Autodesk Inventor part; units mm, degrees
(part 2 of 2)
sketch "草圖23" plane through (-20, 166, 12) normal (0, 0, -1) x (-1, 0, 0)
  line L0 (0, 0) -> (1.75, 0)
  line L1 (9, 0) -> (0, 0) projected
  line L2 (1.75, 0) -> (7.25, 0)
  line L3 (7.25, 0) -> (9, 0)
  line L4 (1.75, 0) -> (7.25, 0)
  line L5 (7.25, 0) -> (7.25, 1)
  line L6 (7.25, 1) -> (1.75, 1)
  line L7 (1.75, 1) -> (1.75, 0)
  line L8 (1.75, 1) -> (7.25, 1)
  line L9 (7.25, 1) -> (7.25, 230)
  line L10 (1.75, 230) -> (1.75, 1)
  line L11 (7.25, 230) -> (7.25, 230.25)
  line L12 (7.25, 230.25) -> (1.75, 230.25)
  line L13 (1.75, 230.25) -> (1.75, 230)
  line L14 (1.75, 230) -> (2, 230)
  line L15 (7.25, 230) -> (7, 230)
  arc A0 (2, 230.25) -> (1.75, 230) centre (2, 230) ccw
  arc A1 (7.25, 230) -> (7, 230.25) centre (7, 230) ccw
  arc A2 (5.2071, 230.25) -> (3.7929, 230.25) centre (4.5, 230) ccw
  line L16 (7.25, 230) -> (5.25, 230)
  line L17 (2.25, 230) -> (1.75, 230)
  line L18 (1.75, 230) -> (3.75, 230)
  line L19 (6.75, 230) -> (7.25, 230)
  point P0 (-20, -166)
  dimension "d366" = 1.75
  dimension "d367" = 5.5
  dimension "d368" = 1
  dimension "d369" = 229
  dimension "d370" = 0.25
  dimension "d371" = 0.25
  dimension "d372" = 0.25
  dimension "d373" = 1.5
  constraints: 38 end point, 10 point on circle, 8 parallel, 8 point on line, 6 collinear, 4 perpendicular, 3 centre point, 2 coincident, 1 horizontal, 1 midpoint, 1 tangent
  measures "d366" distance of L0.start L0.end
  measures "d367" distance of L0.end L2.end
  measures "d368" distance of L5.end L2.end
  measures "d369" distance of L9.end L5.end
  measures "d370" distance of L11.end L9.end
  measures "d371" distance of L10.start L14.end
  measures "d372" distance of L9.end L15.end
  measures "d373" diameter of A2
extrude "擠出20" cut sketch "草圖23" against normal blind 0.6 contours L6 L10 A0 L12 A1 L9 | L12 A2
chamfer "倒角1" distance 3.2 angle 45 8 edges at (-20, 467.5, 28.5) (-20, 484.5, 24.5) (20, 484.5, 24.5) (20, 467.5, 28.5) (-20, 467.5, -28.5) (-20, 484.5, -24.5) (20, 484.5, -24.5) (20, 467.5, -28.5)
sketch "草圖24" plane through (-20, 166, -12) normal (-1, 0, 0) x (0, 0, 1)
  line L0 (0, 0) -> (24, 0) projected
  line L1 (0, 0) -> (0.75, 0)
  line L2 (0.75, 0) -> (6.25, 0)
  line L3 (6.25, 0) -> (9.25, 0)
  line L4 (9.25, 0) -> (14.75, 0)
  line L5 (14.75, 0) -> (17.75, 0)
  line L6 (17.75, 0) -> (23.25, 0)
  line L7 (23.25, 0) -> (24, 0)
  line L8 (-16.5, 313) -> (-12.5, 313) projected
  line L9 (-12.5, 313) -> (36.5, 313)
  line L10 (0.75, 0) -> (6.25, 0)
  line L11 (6.25, 0) -> (6.25, 1)
  line L12 (6.25, 1) -> (0.75, 1)
  line L13 (0.75, 1) -> (0.75, 0)
  line L14 (9.25, 0) -> (14.75, 0)
  line L15 (14.75, 0) -> (14.75, 1)
  line L16 (14.75, 1) -> (9.25, 1)
  line L17 (9.25, 1) -> (9.25, 0)
  line L18 (17.75, 0) -> (23.25, 0)
  line L19 (23.25, 0) -> (23.25, 1)
  line L20 (23.25, 1) -> (17.75, 1)
  line L21 (17.75, 1) -> (17.75, 0)
  line L22 (17.75, 1) -> (23.25, 1)
  line L23 (23.25, 1) -> (23.25, 7)
  line L24 (23.25, 7) -> (17.75, 7)
  line L25 (17.75, 7) -> (17.75, 1)
  line L26 (23.25, 7) -> (17.75, 7)
  line L27 (17.75, 7) -> (17.75, 305)
  line L28 (17.75, 305) -> (23.25, 305)
  line L29 (23.25, 305) -> (23.25, 7)
  arc A0 (23.25, 305) -> (17.75, 305) centre (20.5, 305) ccw
  line L30 (9.25, 1) -> (14.75, 1)
  line L31 (14.75, 1) -> (14.75, 305)
  line L32 (14.75, 305) -> (9.25, 305)
  line L33 (9.25, 305) -> (9.25, 1)
  line L34 (6.25, 1) -> (0.75, 1)
  line L35 (0.75, 1) -> (0.75, 305)
  line L36 (0.75, 305) -> (6.25, 305)
  line L37 (6.25, 305) -> (6.25, 1)
  arc A1 (14.75, 305) -> (9.25, 305) centre (12, 305) ccw
  arc A2 (6.25, 305) -> (0.75, 305) centre (3.5, 305) ccw
  line L38 (26, 290) -> (26.25, 290)
  line L39 (40.5, 290) -> (26, 290) projected
  line L40 (26.25, 290) -> (31.75, 290)
  line L41 (31.75, 290) -> (31.75, 294)
  line L42 (31.75, 294) -> (26.25, 294)
  line L43 (26.25, 294) -> (26.25, 290)
  line L44 (31.75, 294) -> (26.25, 294)
  line L45 (26.25, 294) -> (26.25, 302)
  line L46 (31.75, 302) -> (31.75, 294)
  line L47 (31.75, 302) -> (31.75, 302.25)
  line L48 (26.25, 302.25) -> (26.25, 302)
  line L49 (26.25, 302) -> (26.5, 302)
  line L50 (31.75, 302) -> (31.5, 302)
  arc A3 (26.5, 302.25) -> (26.25, 302) centre (26.5, 302) ccw
  arc A4 (31.75, 302) -> (31.5, 302.25) centre (31.5, 302) ccw
  line L51 (26.25, 302) -> (26.75, 302)
  line L52 (31.25, 302) -> (31.75, 302)
  line L53 (26.25, 302) -> (26.75, 302)
  line L54 (31.25, 302) -> (31.75, 302)
  line L55 (12, 305) -> (12, 299.4398)
  line L56 (-2, 290) -> (-2.25, 290)
  line L57 (-2.25, 290) -> (-7.75, 290)
  line L58 (-7.75, 290) -> (-7.75, 294)
  line L59 (-7.75, 294) -> (-2.25, 294)
  line L60 (-2.25, 294) -> (-2.25, 290)
  line L61 (-7.75, 294) -> (-2.25, 294)
  line L62 (-2.25, 294) -> (-2.25, 302)
  line L63 (-7.75, 302) -> (-7.75, 294)
  line L64 (-7.75, 302) -> (-7.75, 302.25)
  line L65 (-2.25, 302.25) -> (-2.25, 302)
  line L66 (-2.25, 302) -> (-2.5, 302)
  line L67 (-7.75, 302) -> (-7.5, 302)
  arc A5 (-2.25, 302) -> (-2.5, 302.25) centre (-2.5, 302) ccw
  arc A6 (-7.5, 302.25) -> (-7.75, 302) centre (-7.5, 302) ccw
  line L68 (-2.25, 302) -> (-2.75, 302)
  line L69 (-7.25, 302) -> (-7.75, 302)
  line L70 (-2.25, 302) -> (-2.75, 302)
  line L71 (-7.25, 302) -> (-7.75, 302)
  line L72 (31.75, 290) -> (33.3, 290)
  line L73 (33.3, 290) -> (35.8, 290)
  line L74 (37.3, 313) -> (37.3, 290) projected
  line L75 (35.8, 290) -> (37.3, 290)
  line L76 (33.3, 290) -> (35.8, 290)
  line L77 (35.8, 290) -> (35.8, 294)
  line L78 (35.8, 294) -> (33.3, 294)
  line L79 (33.3, 294) -> (33.3, 290)
  line L80 (35.8, 294) -> (33.3, 294)
  line L81 (33.3, 294) -> (33.3, 302)
  line L82 (35.8, 302) -> (35.8, 294)
  line L83 (35.8, 302) -> (35.8, 302.25)
  line L84 (35.8, 302.25) -> (33.3, 302.25)
  line L85 (33.3, 302.25) -> (33.3, 302)
  line L86 (33.3, 302) -> (33.55, 302)
  line L87 (35.8, 302) -> (35.55, 302)
  arc A7 (33.55, 302.25) -> (33.3, 302) centre (33.55, 302) ccw
  arc A8 (35.8, 302) -> (35.55, 302.25) centre (35.55, 302) ccw
  line L88 (33.3, 302) -> (33.8, 302)
  line L89 (35.3, 302) -> (35.8, 302)
  line L90 (33.3, 302) -> (33.8, 302)
  line L91 (35.3, 302) -> (35.8, 302)
  line L92 (-9.3, 290) -> (-11.8, 290)
  line L93 (-9.3, 290) -> (-11.8, 290)
  line L94 (-11.8, 290) -> (-11.8, 294)
  line L95 (-11.8, 294) -> (-9.3, 294)
  line L96 (-9.3, 294) -> (-9.3, 290)
  line L97 (-11.8, 294) -> (-9.3, 294)
  line L98 (-9.3, 294) -> (-9.3, 302)
  line L99 (-11.8, 302) -> (-11.8, 294)
  line L100 (-11.8, 302) -> (-11.8, 302.25)
  line L101 (-11.8, 302.25) -> (-9.3, 302.25)
  line L102 (-9.3, 302.25) -> (-9.3, 302)
  line L103 (-9.3, 302) -> (-9.55, 302)
  line L104 (-11.8, 302) -> (-11.55, 302)
  arc A9 (-9.3, 302) -> (-9.55, 302.25) centre (-9.55, 302) ccw
  arc A10 (-11.55, 302.25) -> (-11.8, 302) centre (-11.55, 302) ccw
  line L105 (-9.3, 302) -> (-9.8, 302)
  line L106 (-11.3, 302) -> (-11.8, 302)
  line L107 (-9.3, 302) -> (-9.8, 302)
  line L108 (-11.3, 302) -> (-11.8, 302)
  arc A11 (29.7071, 302.25) -> (28.2929, 302.25) centre (29, 302) ccw
  line L109 (31.75, 302.25) -> (29.7071, 302.25)
  line L110 (28.2929, 302.25) -> (26.25, 302.25)
  line L111 (26.5, 302) -> (26.75, 302)
  line L112 (31.25, 302) -> (31.5, 302)
  arc A12 (-4.2929, 302.25) -> (-5.7071, 302.25) centre (-5, 302) ccw
  line L113 (-7.75, 302.25) -> (-5.7071, 302.25)
  line L114 (-4.2929, 302.25) -> (-2.25, 302.25)
  line L115 (-7.5, 302) -> (-7.25, 302)
  line L116 (-2.75, 302) -> (-2.5, 302)
  point P0 (12, -166)
  point P1 (28.2502, 302.25)
  point P2 (29.7498, 302.25)
  point P3 (-4.2502, 302.25)
  point P4 (-5.7498, 302.25)
  dimension "d376" = 0.75
  dimension "d377" = 5.5
  dimension "d378" = 3
  dimension "d379" = 5.5
  dimension "d380" = 3
  dimension "d381" = 5.5
  dimension "d382" = 1
  dimension "d383" = 1
  dimension "d384" = 1
  dimension "d385" = 6
  dimension "d386" = 298
  dimension "d387" = 304
  dimension "d388" = 304
  dimension "d389" = 0.25
  dimension "d390" = 5.5
  dimension "d391" = 4
  dimension "d392" = 0.25
  dimension "d393" = 0.25
  dimension "d394" = 0.25
  dimension "d402" = 8
  dimension "d495" = 1.55
  dimension "d496" = 2.5
  dimension "d497" = 4
  dimension "d498" = 8
  dimension "d499" = 0.25
  dimension "d500" = 0.25
  dimension "d501" = 0.25
  dimension "d616" = 1.5
  dimension "d617" = 1.5
  constraints: 226 end point, 35 symmetric about line, 34 point on circle, 32 parallel, 22 point on line, 21 perpendicular, 13 centre point, 12 collinear, 8 coincident, 8 midpoint, 7 tangent, 2 horizontal, 1 vertical, 4 other
  measures "d376" distance of L0.start L1.end
  measures "d377" distance of L1.end L2.end
  measures "d378" distance of L2.end L3.end
  measures "d379" distance of L3.end L4.end
  measures "d380" distance of L4.end L5.end
  measures "d381" distance of L5.end L6.end
  measures "d382" distance of L11.end L2.end
  measures "d383" distance of L15.end L4.end
  measures "d384" distance of L19.end L6.end
  measures "d385" distance of L23.end L19.end
  measures "d386" distance of L24.end L27.end
  measures "d387" distance of L31.end L15.end
  measures "d388" distance of L12.end L35.end
  measures "d389" distance of L38.start L38.end
  measures "d390" distance of L38.end L40.end
  measures "d391" distance of L41.end L40.end
  measures "d392" distance of L46.start L47.end
  measures "d393" distance of L45.end L49.end
  measures "d394" distance of L46.start L50.end
  measures "d402" distance of L46.start L41.end
  measures "d495" distance of L40.end L72.end
  measures "d496" distance of L72.end L73.end
  measures "d497" distance of L77.end L73.end
  measures "d498" distance of L78.end L81.end
  measures "d499" distance of L82.start L83.end
  measures "d500" distance of L81.end L86.end
  measures "d501" distance of L82.start L87.end
  measures "d616" diameter of A11
  measures "d617" diameter of A12
extrude "擠出21" cut sketch "草圖24" against normal blind 0.6 contours L35 L36 L37 L12 | A2 L36 | L33 L32 L31 L16 | A1 L32 | L25 L24 L23 L20 | L27 L28 L29 L24 | A0 L28 | L78 L81 A7 L84 A8 L82 | L42 L45 A3 L110 A11 L109 A4 L46 | A4 L109 L47 | L59 L63 A6 L113 A12 L114 A5 L62 | L64 L113 A6 | L95 L99 A10 L101 A9 L98
sketch "草圖25" plane through (-25, 398, 35) normal (0, 0, 1) x (1, 0, 0)
  line L0 (0, 0) -> (0, 58) projected
  line L1 (3.75, 0) -> (5.25, 0)
  line L2 (5.25, 0) -> (10.75, 0)
  line L3 (10.75, 0) -> (13.75, 0)
  line L4 (13.75, 0) -> (19.25, 0)
  line L5 (19.25, 0) -> (22.25, 0)
  line L6 (22.25, 0) -> (27.75, 0)
  line L7 (27.75, 0) -> (30.75, 0)
  line L8 (30.75, 0) -> (36.25, 0)
  line L9 (36.25, 0) -> (39.25, 0)
  line L10 (39.25, 0) -> (44.75, 0)
  line L11 (44.75, 0) -> (47, 0)
  line L12 (47, 0) -> (49.5, 0)
  line L13 (50, 0) -> (50, 58) projected
  line L14 (49.5, 0) -> (50, 0)
  line L15 (49.5, 0) -> (50, 0)
  line L16 (5.25, 0) -> (3, 0)
  line L17 (5, 73) -> (5, -231) projected
  line L18 (3, 0) -> (0.5, 0)
  line L19 (0.5, 0) -> (0, 0)
  line L20 (0.5, 0) -> (3, 0)
  line L21 (3, 0) -> (3, 1)
  line L22 (3, 1) -> (0.5, 1)
  line L23 (0.5, 1) -> (0.5, 0)
  line L24 (50, 0) -> (0, 0) projected
  line L25 (0.5, 1) -> (3, 1)
  line L26 (3, 1) -> (3, 54)
  line L27 (3, 54) -> (2.5, 54)
  line L28 (0.5, 54) -> (0.5, 1)
  line L29 (0.5, 1) -> (3, 1)
  line L30 (5.25, 0) -> (10.75, 0)
  line L31 (10.75, 0) -> (10.75, 1)
  line L32 (10.75, 1) -> (5.25, 1)
  line L33 (5.25, 1) -> (5.25, 0)
  line L34 (5.25, 1) -> (10.75, 1)
  line L35 (10.75, 1) -> (10.75, 54)
  line L36 (5.25, 54) -> (5.25, 1)
  line L37 (13.75, 0) -> (19.25, 0)
  line L38 (19.25, 0) -> (19.25, 1)
  line L39 (19.25, 1) -> (13.75, 1)
  line L40 (13.75, 1) -> (13.75, 0)
  line L41 (19.25, 1) -> (13.75, 1)
  line L42 (13.75, 1) -> (13.75, 54)
  line L43 (13.75, 54) -> (19.25, 54)
  line L44 (19.25, 54) -> (19.25, 1)
  line L45 (22.25, 0) -> (27.75, 0)
  line L46 (27.75, 0) -> (27.75, 1)
  line L47 (27.75, 1) -> (22.25, 1)
  line L48 (22.25, 1) -> (22.25, 0)
  line L49 (27.75, 1) -> (22.25, 1)
  line L50 (22.25, 1) -> (22.25, 54)
  line L51 (22.25, 54) -> (27.75, 54)
  line L52 (27.75, 54) -> (27.75, 1)
  line L53 (30.75, 0) -> (36.25, 0)
  line L54 (36.25, 0) -> (36.25, 1)
  line L55 (36.25, 1) -> (30.75, 1)
  line L56 (30.75, 1) -> (30.75, 0)
  line L57 (30.75, 1) -> (36.25, 1)
  line L58 (36.25, 1) -> (36.25, 54)
  line L59 (36.25, 54) -> (30.75, 54)
  line L60 (30.75, 54) -> (30.75, 1)
  line L61 (39.25, 0) -> (44.75, 0)
  line L62 (44.75, 0) -> (44.75, 1)
  line L63 (44.75, 1) -> (39.25, 1)
  line L64 (39.25, 1) -> (39.25, 0)
  line L65 (44.75, 1) -> (39.25, 1)
  line L66 (39.25, 1) -> (39.25, 54)
  line L67 (39.25, 54) -> (44.75, 54)
  line L68 (44.75, 54) -> (44.75, 1)
  line L69 (47, 0) -> (49.5, 0)
  line L70 (49.5, 0) -> (49.5, 1)
  line L71 (49.5, 1) -> (47, 1)
  line L72 (47, 1) -> (47, 0)
  line L73 (49.5, 1) -> (47, 1)
  line L74 (47, 1) -> (47, 54)
  line L75 (47, 54) -> (49.5, 54)
  line L76 (49.5, 54) -> (49.5, 1)
  line L77 (10.75, 54) -> (10.75, 54.25)
  line L78 (10.75, 54.25) -> (5.25, 54.25)
  line L79 (5.25, 54.25) -> (5.25, 54)
  line L80 (5.25, 54) -> (5.5, 54)
  line L81 (10.75, 54) -> (10.5, 54)
  arc A0 (5.5, 54.25) -> (5.25, 54) centre (5.5, 54) ccw
  arc A1 (10.75, 54) -> (10.5, 54.25) centre (10.5, 54) ccw
  arc A2 (8.7071, 54.25) -> (7.2929, 54.25) centre (8, 54) ccw
  line L82 (10.75, 54) -> (10.25, 54)
  line L83 (5.75, 54) -> (5.25, 54)
  line L84 (5.25, 54) -> (5.75, 54)
  line L85 (7.25, 54) -> (8.75, 54)
  line L86 (10.25, 54) -> (10.75, 54)
  arc A3 (17.2071, 54.25) -> (15.7929, 54.25) centre (16.5, 54) ccw
  line L87 (19.25, 54.25) -> (13.75, 54.25)
  line L88 (13.75, 54) -> (14, 54)
  arc A4 (14, 54.25) -> (13.75, 54) centre (14, 54) ccw
  arc A5 (19.25, 54) -> (19, 54.25) centre (19, 54) ccw
  line L89 (19.25, 54) -> (19, 54)
  arc A6 (25.7071, 54.25) -> (24.2929, 54.25) centre (25, 54) ccw
  line L90 (27.75, 54.25) -> (22.25, 54.25)
  line L91 (22.25, 54) -> (22.5, 54)
  arc A7 (22.5, 54.25) -> (22.25, 54) centre (22.5, 54) ccw
  arc A8 (27.75, 54) -> (27.5, 54.25) centre (27.5, 54) ccw
  line L92 (27.75, 54) -> (27.5, 54)
  arc A9 (34.2071, 54.25) -> (32.7929, 54.25) centre (33.5, 54) ccw
  line L93 (36.25, 54.25) -> (30.75, 54.25)
  line L94 (30.75, 54) -> (31, 54)
  arc A10 (31, 54.25) -> (30.75, 54) centre (31, 54) ccw
  arc A11 (36.25, 54) -> (36, 54.25) centre (36, 54) ccw
  line L95 (36.25, 54) -> (36, 54)
  arc A12 (42.7071, 54.25) -> (41.2929, 54.25) centre (42, 54) ccw
  line L96 (44.75, 54.25) -> (39.25, 54.25)
  line L97 (39.25, 54) -> (39.5, 54)
  arc A13 (39.5, 54.25) -> (39.25, 54) centre (39.5, 54) ccw
  arc A14 (44.75, 54) -> (44.5, 54.25) centre (44.5, 54) ccw
  line L98 (44.75, 54) -> (44.5, 54)
  line L99 (3, 54) -> (3, 54.25)
  line L100 (3, 54.25) -> (0.5, 54.25)
  line L101 (0.5, 54.25) -> (0.5, 54)
  line L102 (0.5, 54) -> (0.75, 54)
  line L103 (3, 54) -> (2.75, 54)
  arc A15 (0.75, 54.25) -> (0.5, 54) centre (0.75, 54) ccw
  arc A16 (3, 54) -> (2.75, 54.25) centre (2.75, 54) ccw
  line L104 (0.5, 54) -> (1, 54)
  line L105 (2.5, 54) -> (3, 54)
  line L106 (49.5, 54.25) -> (47, 54.25)
  arc A17 (47.25, 54.25) -> (47, 54) centre (47.25, 54) ccw
  arc A18 (49.5, 54) -> (49.25, 54.25) centre (49.25, 54) ccw
  point P0 (25, -398)
  point P1 (5, -231)
  point P2 (15.75, 54)
  point P3 (17.25, 54)
  point P4 (14.25, 54)
  point P5 (18.75, 54)
  point P6 (24.25, 54)
  point P7 (25.75, 54)
  point P8 (22.75, 54)
  point P9 (27.25, 54)
  point P10 (32.75, 54)
  point P11 (34.25, 54)
  point P12 (31.25, 54)
  point P13 (35.75, 54)
  point P14 (41.25, 54)
  point P15 (42.75, 54)
  point P16 (39.75, 54)
  point P17 (44.25, 54)
  point P18 (47.5, 54)
  point P19 (49, 54)
  point P20 (49.5, 54)
  point P21 (47, 54)
  point P22 (39.25, 54)
  point P23 (44.75, 54)
  point P24 (36.25, 54)
  point P25 (30.75, 54)
  point P26 (22.25, 54)
  point P27 (27.75, 54)
  point P28 (13.75, 54)
  point P29 (19.25, 54)
  point P30 (47, 54)
  point P31 (49.5, 54)
  dimension "d408" = 5.5
  dimension "d409" = 3
  dimension "d410" = 5.5
  dimension "d411" = 3
  dimension "d412" = 5.5
  dimension "d413" = 3
  dimension "d414" = 5.5
  dimension "d415" = 3
  dimension "d416" = 5.5
  dimension "d417" = 2.25
  dimension "d418" = 2.5
  dimension "d419" = 2.25
  dimension "d420" = 2.5
  dimension "d421" = 1
  dimension "d422" = 53
  dimension "d428" = 1
  dimension "d429" = 53
  dimension "d430" = 1
  dimension "d431" = 53
  dimension "d432" = 1
  dimension "d433" = 53
  dimension "d434" = 1
  dimension "d435" = 53
  dimension "d436" = 1
  dimension "d437" = 53
  dimension "d438" = 1
  dimension "d439" = 53
  dimension "d440" = 0.25
  dimension "d441" = 0.25
  dimension "d442" = 0.25
  dimension "d443" = 1.5
  dimension "d446" = 8.5
  dimension "d451" = 0.25
  dimension "d452" = 0.25
  dimension "d453" = 0.25
  dimension "d456" = 46.5
  constraints: 206 end point, 62 point on circle, 36 parallel, 36 point on line, 25 perpendicular, 19 centre point, 14 collinear, 12 coincident, 8 horizontal, 5 midpoint, 1 tangent, 105 other
  measures "d408" distance of L1.end L2.end
  measures "d409" distance of L2.end L3.end
  measures "d410" distance of L3.end L4.end
  measures "d411" distance of L4.end L5.end
  measures "d412" distance of L5.end L6.end
  measures "d413" distance of L6.end L7.end
  measures "d414" distance of L7.end L8.end
  measures "d415" distance of L8.end L9.end
  measures "d416" distance of L9.end L10.end
  measures "d417" distance of L10.end L11.end
  measures "d418" distance of L11.end L12.end
  measures "d419" distance of L1.end L16.end
  measures "d420" distance of L16.end L18.end
  measures "d421" distance of L21.end L16.end
  measures "d422" distance of L26.end L21.end
  measures "d428" distance of L31.end L2.end
  measures "d429" distance of L35.end L31.end
  measures "d430" distance of L38.end L4.end
  measures "d431" distance of L39.end L42.end
  measures "d432" distance of L46.end L6.end
  measures "d433" distance of L47.end L50.end
  measures "d434" distance of L54.end L8.end
  measures "d435" distance of L58.end L54.end
  measures "d436" distance of L62.end L10.end
  measures "d437" distance of L63.end L66.end
  measures "d438" distance of L70.end L12.end
  measures "d439" distance of L71.end L74.end
  measures "d440" distance of L77.end L35.end
  measures "d441" distance of L36.start L80.end
  measures "d442" distance of L35.end L81.end
  measures "d443" diameter of A2
  measures "d446" distance of A2.centre A3.centre
  measures "d451" distance of L26.end L99.end
  measures "d452" distance of L28.start L102.end
  measures "d453" distance of L26.end L103.end
  measures "d456" distance of L99.end L106.start
extrude "擠出23" cut sketch "草圖25" against normal blind 0.6 contours L36 A0 L78 A1 L35 L32 | L42 L43 L44 L39 | A4 L87 A5 L43 | A2 L78 | L50 L51 L52 L47 | A7 L90 A8 L51 | A3 L87 | L60 L59 L58 L55 | A10 L93 A11 L59 | A6 L90 | L66 L67 L68 L63 | A13 L96 A14 L67 | A9 L93 | A12 L96
sketch "草圖26" plane through (-25, 398, 14) normal (-1, 0, 0) x (0, 0, 1)
  line L0 (0, 0) -> (0, 58) projected
  line L1 (0, 0) -> (3.25, 0)
  line L2 (21, 0) -> (21, 58) projected
  line L3 (3.25, 0) -> (5.75, 0)
  line L4 (5.75, 0) -> (7, 0)
  line L5 (7, 0) -> (15.5, 0)
  line L6 (15.5, 0) -> (16.75, 0)
  line L7 (16.75, 0) -> (19.25, 0)
  line L8 (19.25, 0) -> (21, 0)
  line L9 (3.25, 0) -> (5.75, 0)
  line L10 (5.75, 0) -> (5.75, 1)
  line L11 (5.75, 1) -> (3.25, 1)
  line L12 (3.25, 1) -> (3.25, 0)
  line L13 (24, 0) -> (-2, 0) projected
  line L14 (5.75, 1) -> (3.25, 1)
  line L15 (3.25, 1) -> (3.25, 54)
  line L16 (5.75, 54) -> (5.75, 1)
  line L17 (7, 0) -> (15.5, 0)
  line L18 (15.5, 0) -> (15.5, 1)
  line L19 (15.5, 1) -> (7, 1)
  line L20 (7, 1) -> (7, 0)
  line L21 (15.5, 1) -> (7, 1)
  line L22 (7, 1) -> (7, 54)
  line L23 (7, 54) -> (15.5, 54)
  line L24 (15.5, 54) -> (15.5, 1)
  line L25 (16.75, 0) -> (19.25, 0)
  line L26 (19.25, 0) -> (19.25, 1)
  line L27 (19.25, 1) -> (16.75, 1)
  line L28 (16.75, 1) -> (16.75, 0)
  line L29 (19.25, 1) -> (16.75, 1)
  line L30 (16.75, 1) -> (16.75, 54)
  line L31 (16.75, 54) -> (19.25, 54)
  line L32 (19.25, 54) -> (19.25, 1)
  line L33 (5.75, 54) -> (5.75, 54.25)
  line L34 (5.75, 54.25) -> (3.25, 54.25)
  line L35 (3.25, 54.25) -> (3.25, 54)
  line L36 (3.25, 54) -> (3.5, 54)
  line L37 (5.75, 54) -> (5.5, 54)
  arc A0 (3.5, 54.25) -> (3.25, 54) centre (3.5, 54) ccw
  arc A1 (5.75, 54) -> (5.5, 54.25) centre (5.5, 54) ccw
  line L38 (3.25, 54) -> (3.75, 54)
  line L39 (5.25, 54) -> (5.75, 54)
  line L40 (3.25, 54) -> (3.75, 54)
  line L41 (5.25, 54) -> (5.75, 54)
  arc A2 (17, 54.25) -> (16.75, 54) centre (17, 54) ccw
  line L42 (19.25, 54.25) -> (16.75, 54.25)
  arc A3 (19.25, 54) -> (19, 54.25) centre (19, 54) ccw
  line L43 (7, 54) -> (15.5, 54)
  line L44 (15.5, 54) -> (15.5, 54.25)
  line L45 (15.5, 54.25) -> (7, 54.25)
  line L46 (7, 54.25) -> (7, 54)
  line L47 (7, 54) -> (7.25, 54)
  line L48 (15.5, 54) -> (15.25, 54)
  arc A4 (7.25, 54.25) -> (7, 54) centre (7.25, 54) ccw
  arc A5 (15.5, 54) -> (15.25, 54.25) centre (15.25, 54) ccw
  line L49 (7.25, 54) -> (9.75, 54)
  line L50 (15.25, 54) -> (12.75, 54)
  arc A6 (10.4571, 54.25) -> (9.0429, 54.25) centre (9.75, 54) ccw
  arc A7 (13.4571, 54.25) -> (12.0429, 54.25) centre (12.75, 54) ccw
  point P0 (-14, -398)
  point P1 (17.25, 54)
  point P2 (18.75, 54)
  point P3 (19.25, 54)
  point P4 (16.75, 54)
  dimension "d461" = 3.25
  dimension "d462" = 2.5
  dimension "d463" = 1.25
  dimension "d464" = 8.5
  dimension "d465" = 1.25
  dimension "d466" = 2.5
  dimension "d467" = 1.75
  dimension "d468" = 1
  dimension "d469" = 53
  dimension "d470" = 1
  dimension "d471" = 53
  dimension "d472" = 1
  dimension "d473" = 53
  dimension "d474" = 0.25
  dimension "d475" = 0.25
  dimension "d476" = 0.25
  dimension "d479" = 13.5
  dimension "d484" = 0.25
  dimension "d485" = 0.25
  dimension "d486" = 0.25
  dimension "d487" = 2.5
  dimension "d488" = 2.5
  dimension "d489" = 1.5
  dimension "d490" = 1.5
  constraints: 96 end point, 20 point on circle, 20 point on line, 18 parallel, 11 perpendicular, 9 collinear, 8 centre point, 6 coincident, 3 horizontal, 2 midpoint, 13 other
  measures "d461" distance of L0.start L1.end
  measures "d462" distance of L1.end L3.end
  measures "d463" distance of L3.end L4.end
  measures "d464" distance of L4.end L5.end
  measures "d465" distance of L5.end L6.end
  measures "d466" distance of L6.end L7.end
  measures "d467" distance of L7.end L8.end
  measures "d468" distance of L10.end L3.end
  measures "d469" distance of L11.end L15.end
  measures "d470" distance of L18.end L5.end
  measures "d471" distance of L22.end L19.end
  measures "d472" distance of L26.end L7.end
  measures "d473" distance of L27.end L30.end
  measures "d474" distance of L33.end L16.start
  measures "d475" distance of L15.end L36.end
  measures "d476" distance of L16.start L37.end
  measures "d479" distance of A0.centre A2.centre
  measures "d484" distance of L44.end L23.end
  measures "d485" distance of L22.end L47.end
  measures "d486" distance of L23.end L48.end
  measures "d487" distance of L49.start L49.end
  measures "d488" distance of L50.start L50.end
  measures "d489" diameter of A6
  measures "d490" diameter of A7
extrude "擠出24" cut sketch "草圖26" against normal blind 0.6 contours L15 A0 L34 A1 L16 L11 | L22 L23 L24 L19 | A4 L45 A5 L23 | L30 L31 L32 L27 | A2 L42 A3 L31 | A6 L45 | L45 A7
ref_plane "工作平面6" through (-25, 398, 24.5) normal (0, 0, 1) x (1, 0, 0)
extrude "擠出25" cut sketch "草圖25" against normal blind 0.6 contours L22 L28 A15 L100 A16 L26 | L74 L75 L76 L71 | A17 L106 A18 L75
sketch "草圖27" plane through (-16.8, 479, 28.5) normal (0, 0, 1) x (1, 0, 0)
  line L0 (33.6, 0) -> (33.6, -23) projected
  line L1 (0, -23) -> (0.1, -23)
  line L2 (2.55, -27) -> (2.55, -80) projected
  line L3 (33.6, -23) -> (0, -23) projected
  line L4 (2.55, -23) -> (0.05, -23)
  line L5 (0.05, -23) -> (0, -23)
  line L6 (2.55, -23) -> (5.55, -23)
  line L7 (5.55, -23) -> (11.05, -23)
  line L8 (11.05, -23) -> (14.05, -23)
  line L9 (14.05, -23) -> (19.55, -23)
  line L10 (19.55, -23) -> (22.55, -23)
  line L11 (22.55, -23) -> (28.05, -23)
  line L12 (28.05, -23) -> (31.05, -23)
  line L13 (31.05, -23) -> (33.55, -23)
  line L14 (33.55, -23) -> (33.6, -23)
  line L15 (2.55, -23) -> (0.05, -23)
  line L16 (0.05, -23) -> (0.05, -19)
  line L17 (0.05, -19) -> (2.55, -19)
  line L18 (2.55, -19) -> (2.55, -23)
  line L19 (5.55, -23) -> (11.05, -23)
  line L20 (11.05, -23) -> (11.05, -19)
  line L21 (11.05, -19) -> (5.55, -19)
  line L22 (5.55, -19) -> (5.55, -23)
  line L23 (11.05, -19) -> (5.55, -19)
  line L24 (5.55, -19) -> (5.55, -11)
  line L25 (11.05, -11) -> (11.05, -19)
  line L26 (14.05, -23) -> (19.55, -23)
  line L27 (19.55, -23) -> (19.55, -19)
  line L28 (19.55, -19) -> (14.05, -19)
  line L29 (14.05, -19) -> (14.05, -23)
  line L30 (19.55, -19) -> (14.05, -19)
  line L31 (14.05, -19) -> (14.05, -11)
  line L32 (14.05, -11) -> (19.55, -11)
  line L33 (19.55, -11) -> (19.55, -19)
  line L34 (22.55, -23) -> (28.05, -23)
  line L35 (28.05, -23) -> (28.05, -19)
  line L36 (28.05, -19) -> (22.55, -19)
  line L37 (22.55, -19) -> (22.55, -23)
  line L38 (28.05, -19) -> (22.55, -19)
  line L39 (22.55, -19) -> (22.55, -11)
  line L40 (22.55, -11) -> (28.05, -11)
  line L41 (28.05, -11) -> (28.05, -19)
  line L42 (31.05, -23) -> (33.55, -23)
  line L43 (33.55, -23) -> (33.55, -19)
  line L44 (33.55, -19) -> (31.05, -19)
  line L45 (31.05, -19) -> (31.05, -23)
  line L46 (33.55, -19) -> (31.05, -19)
  line L47 (31.05, -19) -> (31.05, -11)
  line L48 (31.05, -11) -> (33.55, -11)
  line L49 (33.55, -11) -> (33.55, -19)
  line L50 (2.55, -19) -> (0.05, -19)
  line L51 (0.05, -19) -> (0.05, -11)
  line L52 (2.55, -11) -> (2.55, -19)
  line L53 (2.55, -11) -> (0.05, -11)
  line L54 (0.05, -11) -> (0.05, -10.75)
  line L55 (0.05, -10.75) -> (2.55, -10.75)
  line L56 (2.55, -10.75) -> (2.55, -11)
  line L57 (5.55, -11) -> (11.05, -11)
  line L58 (11.05, -11) -> (11.05, -10.75)
  line L59 (11.05, -10.75) -> (5.55, -10.75)
  line L60 (5.55, -10.75) -> (5.55, -11)
  line L61 (0.05, -10.75) -> (0.3, -10.75)
  line L62 (2.55, -10.75) -> (2.3, -10.75)
  line L63 (5.55, -10.75) -> (5.8, -10.75)
  line L64 (11.05, -10.75) -> (10.8, -10.75)
  arc A0 (0.3, -10.75) -> (0.05, -11) centre (0.3, -11) ccw
  arc A1 (2.55, -11) -> (2.3, -10.75) centre (2.3, -11) ccw
  arc A2 (5.8, -10.75) -> (5.55, -11) centre (5.8, -11) ccw
  arc A3 (11.05, -11) -> (10.8, -10.75) centre (10.8, -11) ccw
  line L65 (0.05, -11) -> (0.55, -11)
  line L66 (2.05, -11) -> (2.55, -11)
  line L67 (31.05, -10.75) -> (33.55, -10.75)
  arc A4 (31.3, -10.75) -> (31.05, -11) centre (31.3, -11) ccw
  arc A5 (33.55, -11) -> (33.3, -10.75) centre (33.3, -11) ccw
  arc A6 (9.0071, -10.75) -> (7.5929, -10.75) centre (8.3, -11) ccw
  line L68 (5.55, -11) -> (6.05, -11)
  line L69 (10.55, -11) -> (11.05, -11)
  arc A7 (17.5071, -10.75) -> (16.0929, -10.75) centre (16.8, -11) ccw
  line L70 (19.55, -10.75) -> (14.05, -10.75)
  line L71 (14.05, -10.75) -> (14.3, -10.75)
  arc A8 (14.3, -10.75) -> (14.05, -11) centre (14.3, -11) ccw
  arc A9 (19.55, -11) -> (19.3, -10.75) centre (19.3, -11) ccw
  line L72 (19.05, -11) -> (19.55, -11)
  arc A10 (26.0071, -10.75) -> (24.5929, -10.75) centre (25.3, -11) ccw
  line L73 (28.05, -10.75) -> (22.55, -10.75)
  line L74 (22.55, -10.75) -> (22.8, -10.75)
  arc A11 (22.8, -10.75) -> (22.55, -11) centre (22.8, -11) ccw
  arc A12 (28.05, -11) -> (27.8, -10.75) centre (27.8, -11) ccw
  line L75 (27.55, -11) -> (28.05, -11)
  point P0 (16.8, -479)
  point P1 (33.55, -11)
  point P2 (31.05, -11)
  point P3 (22.55, -11)
  point P4 (28.05, -11)
  point P5 (14.05, -11)
  point P6 (19.55, -11)
  dimension "d505" = 0.1
  dimension "d507" = 2.5
  dimension "d508" = 3
  dimension "d509" = 5.5
  dimension "d510" = 3
  dimension "d511" = 5.5
  dimension "d512" = 3
  dimension "d513" = 5.5
  dimension "d514" = 3
  dimension "d515" = 2.5
  dimension "d516" = 4
  dimension "d517" = 4
  dimension "d518" = 8
  dimension "d519" = 4
  dimension "d520" = 8
  dimension "d521" = 4
  dimension "d522" = 8
  dimension "d523" = 4
  dimension "d524" = 8
  dimension "d525" = 8
  dimension "d526" = 0.25
  dimension "d527" = 0.25
  dimension "d528" = 0.25
  dimension "d529" = 0.25
  dimension "d530" = 0.25
  dimension "d531" = 0.25
  dimension "d535" = 31
  dimension "d542" = 8.5
  constraints: 146 end point, 26 parallel, 26 point on circle, 20 point on line, 17 perpendicular, 13 centre point, 11 collinear, 4 horizontal, 1 midpoint, 56 other
  measures "d505" distance of L1.start L1.end
  measures "d507" distance of L4.start L4.end
  measures "d508" distance of L4.start L6.end
  measures "d509" distance of L6.end L7.end
  measures "d510" distance of L7.end L8.end
  measures "d511" distance of L8.end L9.end
  measures "d512" distance of L9.end L10.end
  measures "d513" distance of L10.end L11.end
  measures "d514" distance of L11.end L12.end
  measures "d515" distance of L12.end L13.end
  measures "d516" distance of L4.end L16.end
  measures "d517" distance of L20.end L7.end
  measures "d518" distance of L21.end L24.end
  measures "d519" distance of L27.end L9.end
  measures "d520" distance of L28.end L31.end
  measures "d521" distance of L35.end L11.end
  measures "d522" distance of L36.end L39.end
  measures "d523" distance of L43.end L13.end
  measures "d524" distance of L44.end L47.end
  measures "d525" distance of L51.end L16.end
  measures "d526" distance of L51.end L54.end
  measures "d527" distance of L25.start L58.end
  measures "d528" distance of L54.end L61.end
  measures "d529" distance of L55.end L62.end
  measures "d530" distance of L63.end L59.end
  measures "d531" distance of L58.end L64.end
  measures "d535" distance of L54.end L67.start
  measures "d542" distance of A6.centre A7.centre
extrude "擠出26" cut sketch "草圖27" against normal blind 0.6 contours L51 L53 L52 L17 | L24 L57 L25 L21 | A2 L59 A3 L57 | L31 L32 L33 L28 | A8 L70 A9 L32 | A6 L59 | L39 L40 L41 L36 | A11 L73 A12 L40 | A7 L70 | L47 L48 L49 L44 | A4 L67 A5 L48 | A10 L73
mirror "鏡射7" about plane through (-25, 398, 24.5) normal (0, 0, 1) of "擠出25"
mirror "鏡射8" about plane through (-22, 166, 0) normal (0, 0, 1) of "擠出12", "擠出14", "擠出15", "擠出16", "擠出18", "擠出19", "擠出20", "擠出24", "擠出23", "擠出26", "擠出25", "鏡射7", "擠出17"
mirror "鏡射9" about plane through (0, 0, -55) normal (-1, 0, 0) of "擠出21", "擠出20", "擠出24", "擠出19", "擠出13", "擠出15", "擠出12", "擠出14", "擠出16", "擠出18", "擠出23", "擠出26", "擠出25", "鏡射8", "鏡射7", "擠出17"
sketch "草圖28" plane through (-29, 0, -20) normal (-1, 0, 0) x (0, 0, 1)
  point P0 (20, 0)
sketch "草圖29" plane through (-20, 166, -12) normal (-1, 0, 0) x (0, 0, 1)
  point P0 (12, -166)
sketch "草圖30" plane through (28, 0, -71) normal (0, 0, -1) x (-1, 0, 0)
  line L0 (0, 0) -> (56, 0) projected
  line L1 (30.75, 0) -> (33.75, 0)
  line L2 (33.75, 0) -> (39.25, 0)
  line L3 (39.25, 0) -> (41.25, 0)
  line L4 (41.25, 0) -> (46.75, 0)
  line L5 (46.75, 0) -> (48.75, 0)
  line L6 (48.75, 0) -> (54.25, 0)
  line L7 (25.25, 0) -> (22.25, 0)
  line L8 (22.25, 0) -> (16.75, 0)
  line L9 (16.75, 0) -> (14.75, 0)
  line L10 (14.75, 0) -> (9.25, 0)
  line L11 (9.25, 0) -> (7.25, 0)
  line L12 (7.25, 0) -> (1.75, 0)
  line L13 (1.75, 0) -> (0, 0)
  line L14 (25.25, 0) -> (30.75, 0)
  line L15 (25.25, 0) -> (30.75, 0)
  line L16 (1.75, 0) -> (7.25, 0)
  line L17 (7.25, 0) -> (7.25, 4)
  line L18 (7.25, 4) -> (1.75, 4)
  line L19 (1.75, 4) -> (1.75, 0)
  line L20 (9.25, 0) -> (14.75, 0)
  line L21 (14.75, 0) -> (14.75, 4)
  line L22 (14.75, 4) -> (9.25, 4)
  line L23 (9.25, 4) -> (9.25, 0)
  line L24 (16.75, 0) -> (22.25, 0)
  line L25 (22.25, 0) -> (22.25, 4)
  line L26 (22.25, 4) -> (16.75, 4)
  line L27 (16.75, 4) -> (16.75, 0)
  line L28 (25.25, 0) -> (30.75, 0)
  line L29 (30.75, 0) -> (30.75, 4)
  line L30 (30.75, 4) -> (25.25, 4)
  line L31 (25.25, 4) -> (25.25, 0)
  line L32 (33.75, 0) -> (39.25, 0)
  line L33 (39.25, 0) -> (39.25, 4)
  line L34 (39.25, 4) -> (33.75, 4)
  line L35 (33.75, 4) -> (33.75, 0)
  line L36 (41.25, 0) -> (46.75, 0)
  line L37 (46.75, 0) -> (46.75, 4)
  line L38 (46.75, 4) -> (41.25, 4)
  line L39 (41.25, 4) -> (41.25, 0)
  line L40 (48.75, 0) -> (54.25, 0)
  line L41 (54.25, 0) -> (54.25, 4)
  line L42 (54.25, 4) -> (48.75, 4)
  line L43 (48.75, 4) -> (48.75, 0)
  line L44 (1.75, 4) -> (7.25, 4)
  line L45 (7.25, 4) -> (7.25, 84)
  line L46 (1.75, 84) -> (1.75, 4)
  line L47 (9.25, 4) -> (14.75, 4)
  line L48 (14.75, 4) -> (14.75, 84)
  line L49 (14.75, 84) -> (9.25, 84)
  line L50 (9.25, 84) -> (9.25, 4)
  line L51 (16.75, 4) -> (22.25, 4)
  line L52 (22.25, 4) -> (22.25, 84)
  line L53 (22.25, 84) -> (16.75, 84)
  line L54 (16.75, 84) -> (16.75, 4)
  line L55 (25.25, 4) -> (30.75, 4)
  line L56 (30.75, 4) -> (30.75, 84)
  line L57 (30.75, 84) -> (25.25, 84)
  line L58 (25.25, 84) -> (25.25, 4)
  line L59 (7.25, 84) -> (7.25, 84.25)
  line L60 (7.25, 84.25) -> (1.75, 84.25)
  line L61 (1.75, 84.25) -> (1.75, 84)
  line L62 (1.75, 84) -> (2, 84)
  line L63 (7.25, 84) -> (7, 84)
  arc A0 (2, 84.25) -> (1.75, 84) centre (2, 84) ccw
  arc A1 (7.25, 84) -> (7, 84.25) centre (7, 84) ccw
  arc A2 (5.2071, 84.25) -> (3.7929, 84.25) centre (4.5, 84) ccw
  line L64 (7.25, 84) -> (6.75, 84)
  line L65 (2.25, 84) -> (1.75, 84)
  line L66 (6.75, 84) -> (7.25, 84)
  line L67 (1.75, 84) -> (2.25, 84)
  arc A3 (12.7071, 84.25) -> (11.2929, 84.25) centre (12, 84) ccw
  line L68 (14.75, 84.25) -> (9.25, 84.25)
  arc A4 (14.75, 84) -> (14.5, 84.25) centre (14.5, 84) ccw
  arc A5 (9.5, 84.25) -> (9.25, 84) centre (9.5, 84) ccw
  arc A6 (20.2071, 84.25) -> (18.7929, 84.25) centre (19.5, 84) ccw
  line L69 (22.25, 84.25) -> (16.75, 84.25)
  arc A7 (22.25, 84) -> (22, 84.25) centre (22, 84) ccw
  arc A8 (17, 84.25) -> (16.75, 84) centre (17, 84) ccw
  arc A9 (25.5, 84.25) -> (25.25, 84) centre (25.5, 84) ccw
  arc A10 (28.7071, 84.25) -> (27.2929, 84.25) centre (28, 84) ccw
  line L70 (30.75, 84.25) -> (25.25, 84.25)
  arc A11 (30.75, 84) -> (30.5, 84.25) centre (30.5, 84) ccw
  point P0 (28, 0)
  point P1 (14.25, 84)
  point P2 (9.75, 84)
  point P3 (21.75, 84)
  point P4 (17.25, 84)
  point P5 (25.75, 84)
  point P6 (30.25, 84)
  point P7 (25.25, 84)
  point P8 (9.25, 84)
  dimension "d550" = 3
  dimension "d551" = 5.5
  dimension "d552" = 2
  dimension "d553" = 5.5
  dimension "d554" = 2
  dimension "d555" = 5.5
  dimension "d557" = 3
  dimension "d558" = 5.5
  dimension "d559" = 2
  dimension "d560" = 5.5
  dimension "d561" = 2
  dimension "d562" = 5.5
  dimension "d563" = 5.5
  dimension "d564" = 4
  dimension "d565" = 4
  dimension "d566" = 4
  dimension "d567" = 4
  dimension "d568" = 4
  dimension "d569" = 4
  dimension "d570" = 4
  dimension "d571" = 80
  dimension "d572" = 80
  dimension "d573" = 80
  dimension "d574" = 80
  dimension "d575" = 0.25
  dimension "d576" = 0.25
  dimension "d577" = 0.25
  dimension "d581" = 7.5
  dimension "d588" = 8.5
  constraints: 140 end point, 32 point on circle, 26 parallel, 16 point on line, 14 perpendicular, 12 centre point, 10 collinear, 10 horizontal, 6 coincident, 2 midpoint, 68 other
  measures "d550" distance of L1.start L1.end
  measures "d551" distance of L1.end L2.end
  measures "d552" distance of L2.end L3.end
  measures "d553" distance of L3.end L4.end
  measures "d554" distance of L4.end L5.end
  measures "d555" distance of L5.end L6.end
  measures "d557" distance of L7.start L7.end
  measures "d558" distance of L7.end L8.end
  measures "d559" distance of L8.end L9.end
  measures "d560" distance of L9.end L10.end
  measures "d561" distance of L10.end L11.end
  measures "d562" distance of L11.end L12.end
  measures "d563" distance of L7.start L1.start
  measures "d564" distance of L17.end L11.end
  measures "d565" distance of L21.end L9.end
  measures "d566" distance of L25.end L7.end
  measures "d567" distance of L29.end L1.start
  measures "d568" distance of L33.end L2.end
  measures "d569" distance of L37.end L4.end
  measures "d570" distance of L41.end L6.end
  measures "d571" distance of L45.end L17.end
  measures "d572" distance of L48.end L21.end
  measures "d573" distance of L52.end L25.end
  measures "d574" distance of L56.end L29.end
  measures "d575" distance of L59.end L45.end
  measures "d576" distance of L46.start L62.end
  measures "d577" distance of L45.end L63.end
  measures "d581" distance of A2.centre A3.centre
  measures "d588" distance of A8.centre A9.centre
extrude "擠出27" cut sketch "草圖30" against normal blind 0.6 contours L46 A0 L60 A1 L45 L18 | L50 L49 L48 L22 | A5 L68 A4 L49 | A2 L60 | L54 L53 L52 L26 | A8 L69 A7 L53 | A3 L68 | L58 L57 L56 L30 | A9 L70 A11 L57 | A6 L69 | A10 L70
mirror "鏡射10" about plane through (0, 0, -55) normal (-1, 0, 0) of "擠出27"
mirror "鏡射11" about plane through (-22, 166, 0) normal (0, 0, 1) of "擠出27", "鏡射10"
sketch "草圖31" plane through (28, 0, -55) normal (1, 0, 0) x (0, 0, -1)
  line L0 (-35, 0) -> (0, 0) projected
  line L1 (0, 0) -> (0.5, 0)
  line L2 (16, 0) -> (16, 86) projected
  line L3 (0.5, 0) -> (6, 0)
  line L4 (6, 0) -> (8, 0)
  line L5 (8, 0) -> (13.5, 0)
  line L6 (13.5, 0) -> (16, 0)
  line L7 (0.5, 0) -> (6, 0)
  line L8 (6, 0) -> (6, 4)
  line L9 (6, 4) -> (0.5, 4)
  line L10 (0.5, 4) -> (0.5, 0)
  line L11 (8, 0) -> (13.5, 0)
  line L12 (13.5, 0) -> (13.5, 4)
  line L13 (13.5, 4) -> (8, 4)
  line L14 (8, 4) -> (8, 0)
  line L15 (0.5, 4) -> (6, 4)
  line L16 (6, 4) -> (6, 84)
  line L17 (6, 84) -> (0.5, 84)
  line L18 (0.5, 84) -> (0.5, 4)
  line L19 (8, 4) -> (13.5, 4)
  line L20 (13.5, 4) -> (13.5, 84)
  line L21 (8, 84) -> (8, 4)
  line L22 (13.5, 84) -> (13.5, 84.25)
  line L23 (8, 84.25) -> (8, 84)
  line L24 (8, 84) -> (8.25, 84)
  line L25 (13.5, 84) -> (13.25, 84)
  arc A0 (8.25, 84.25) -> (8, 84) centre (8.25, 84) ccw
  arc A1 (13.5, 84) -> (13.25, 84.25) centre (13.25, 84) ccw
  arc A2 (11.4571, 84.25) -> (10.0429, 84.25) centre (10.75, 84) ccw
  line L26 (13.5, 84) -> (13, 84)
  line L27 (8, 84) -> (8.5, 84)
  line L28 (13, 84) -> (13.5, 84)
  line L29 (8.5, 84) -> (8, 84)
  line L30 (13.5, 84.25) -> (11.4571, 84.25)
  line L31 (10.0429, 84.25) -> (8, 84.25)
  arc A3 (6, 84) -> (5.75, 84.25) centre (5.75, 84) ccw
  line L32 (2.5429, 84.25) -> (0.5, 84.25)
  line L33 (0.5, 84) -> (1, 84)
  arc A4 (3.9571, 84.25) -> (2.5429, 84.25) centre (3.25, 84) ccw
  line L34 (6, 84.25) -> (3.9571, 84.25)
  arc A5 (0.75, 84.25) -> (1, 84) centre (0.75, 84) ccw
  point P0 (-55, 0)
  point P1 (5.5, 84)
  point P2 (0.5, 84)
  point P3 (6, 84)
  dimension "d595" = 0.5
  dimension "d596" = 5.5
  dimension "d597" = 2
  dimension "d598" = 5.5
  dimension "d599" = 4
  dimension "d600" = 4
  dimension "d601" = 80
  dimension "d602" = 80
  dimension "d603" = 0.25
  dimension "d604" = 0.25
  dimension "d605" = 0.25
  dimension "d609" = 7.5
  constraints: 66 end point, 15 point on circle, 14 parallel, 9 collinear, 8 perpendicular, 8 point on line, 6 centre point, 3 coincident, 3 midpoint, 1 horizontal, 17 other
  measures "d595" distance of L0.end L1.end
  measures "d596" distance of L1.end L3.end
  measures "d597" distance of L3.end L4.end
  measures "d598" distance of L4.end L5.end
  measures "d599" distance of L8.end L3.end
  measures "d600" distance of L12.end L5.end
  measures "d601" distance of L16.end L8.end
  measures "d602" distance of L20.end L12.end
  measures "d603" distance of L20.end L22.end
  measures "d604" distance of L21.start L24.end
  measures "d605" distance of L20.end L25.end
  measures "d609" distance of A1.centre A3.centre
extrude "擠出28" cut sketch "草圖31" against normal blind 0.6 contours L18 A5 L17 L16 L9 | A5 L32 A4 L34 A3 L17 | L17 A5 | L21 A0 L31 A2 L30 A1 L20 L13
mirror "鏡射12" about plane through (0, 0, -55) normal (-1, 0, 0) of "擠出28"
mirror "鏡射13" about plane through (-22, 166, 0) normal (0, 0, 1) of "擠出28", "鏡射12"
